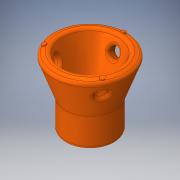
# Autodesk Inventor part: centralLineSplitter
Saved by Autodesk Inventor 2016 (Build 200138000, 138)
## iProperties
Created: 2015-10-15
Part Number: centralLineSplitter
Material: Phenolic Resin
Document SubType Name: Modeling
Designer: ddeboer
Density: 1.38 g/cm^3
Appearance: Smooth - Light Orange
Mass: 152.736 g
Surface Area: 224.412 cm^2
Volume: 110.678 cm^3
Author: ddeboer
Autodesk Inventor part; units mm, degrees
ref_plane "YZ Plane" through (0, 0, 0) normal (1, 0, 0) x (0, 1, 0)
sketch "Sketch1" plane through (0, 0, 0) normal (0, 0, 1) x (1, 0, 0)
  line L0 (0, -30) -> (24.992, -30)
  line L1 (24.992, -30) -> (24.992, -0.6322)
  line L2 (14.5803, 0) -> (0, 0)
  line L3 (0, 0) -> (0, -30)
  line L4 (24.992, -0.6322) -> (38.6728, 36.9555)
  line L5 (24.992, -0.6322) -> (64.992, -0.6322) construction
  line L6 (29.2759, 40.3757) -> (14.5803, 0)
  line L7 (0, -44.0751) -> (0, 54.4509) projected
  line L8 (29.2759, 40.3757) -> (38.6728, 36.9555)
  dimension "d0" = 25
  dimension "d1" = 30
  dimension "d2" = 40
  dimension "d3" = 70
  dimension "d4" = 10
  constraints: 17 end point, 3 parallel, 2 horizontal, 2 perpendicular, 1 coincident
  measures "d0" distance of L2.end L1.end
  measures "d1" distance of L2.end L0.start
  measures "d2" distance of L1.end L4.end
  measures "d3" angle of L5 L4
  measures "d4" distance of L4.end L6.start
revolve "Revolution1" add sketch "Sketch1" angle 360 about axis through (0, -10, 0) along (0, 1, 0)
sketch "Sketch2" plane through (0, -30, 0) normal (0, -1, 0) x (1, 0, 0)
  circle A0 centre (0, 0) radius 5
  dimension "d6" = 10
  constraints: 1 centre point, 1 coincident
  measures "d6" diameter of A0
extrude "Extrusion1" cut sketch "Sketch2" against normal through all
sketch "Sketch3" plane through (0, 0, 0) normal (0, 1, 0) x (1, 0, 0)
  circle A0 centre (0, 0) radius 10
  dimension "d9" = 20
  constraints: 1 centre point, 1 coincident
  measures "d9" diameter of A0
extrude "Extrusion2" cut sketch "Sketch3" against normal blind 10
sketch "Sketch6" plane through (0, -30, 0) normal (0, -1, 0) x (1, 0, 0)
  circle A0 centre (0, 0) radius 24.992 projected
  point P0 (0, -24.992)
  constraints: 1 vertical alignment, 1 other
ref_plane "Work Plane1" through (0, -30, -24.992) normal (0, 0, -1) x (-1, 0, 0)
sketch "Sketch8" plane through (0, -30, -24.992) normal (0, 0, -1) x (-1, 0, 0)
  line L0 (-24.992, 0) -> (24.992, 0) projected
  line L1 (-10.9261, 0) -> (10.8408, 0)
  point P0 (0, 30)
  constraints: 2 end point, 2 point on line
ref_plane "Work Plane2" through (24.992, -30, -24.992) normal (0, -0.258819, -0.9659258) x (-1, 0, 0)
sketch "Sketch9" plane through (24.992, -30, -24.992) normal (0, -0.258819, -0.9659258) x (-1, 0, 0)
  circle A0 centre (24.992, 53.5316) radius 5
  ellipse E0 centre (24.992, -6.4684) end of major axis (0, -6.4684) minor radius 6.4684 projected
  point P0 (24.992, 22.5094)
  dimension "d13" = 10
  dimension "d14" = 60
  constraints: 1 centre point, 1 other
  measures "d13" diameter of A0
  measures "d14" distance of A0.centre point (24.992, -6.468)
extrude "Extrusion3" cut sketch "Sketch9" against normal blind 20 contours A0
pattern_circular "Circular Pattern1" count 3 over 360 about axis through (0, -10, 0) along (0, 1, 0) of "Extrusion3"
fillet "Fillet3" radius 3.175 6 edges at (-22.8009, 25.7946, 7.3908) (4.9998, 25.7946, -23.4415) (26.323, 23.1702, 20.971) (17.801, 25.7946, 16.0508) (-31.3229, 23.1702, 12.3109) (4.9999, 23.1702, -33.2819)
fillet "Fillet6" radius 3.175 3 edges at (-5, -30, 0) (-10, 0, 0) (-5, -10, 0)
fillet "Fillet7" radius 3.175 1 edges at (-24.992, -30, 0)
ref_plane "Work Plane4" through (0, 38.5, 0) normal (0, 1, 0) x (-1, 0, 0)
sketch "Sketch12" plane through (0, 38.5, 0) normal (0, 1, 0) x (-1, 0, 0)
  circle A0 centre (0, 0) radius 38.6728 projected
  line L0 (0, -38.6728) -> (-20.7244, -38.6728)
  constraints: 2 end point, 2 horizontal, 1 vertical alignment, 1 other
ref_plane "Work Plane5" through (0, 38.5, -38.6728) normal (0, 0.9659258, -0.258819) x (1, 0, 0)
sketch "Sketch13" plane through (0, 38.5, -38.6728) normal (0, 0.9659258, -0.258819) x (1, 0, 0)
  circle A0 centre (0, -4.5305) radius 2.2328
  point P0 (0, -27.3905)
  dimension "d31" = 22.86
  constraints: 1 centre point
  measures "d31" distance of A0.centre point (0, -27.391)
extrude "Extrusion4" add sketch "Sketch13" against normal blind 2.54
fillet "Fillet8" radius 3.175 2 edges at (-29.2759, 40.3757, 0) (-38.6728, 36.9555, 0)
pattern_circular "Circular Pattern2" count 3 over 360 about axis through (0, -10, 0) along (0, 1, 0) of "Extrusion4"
body "Solid1"
